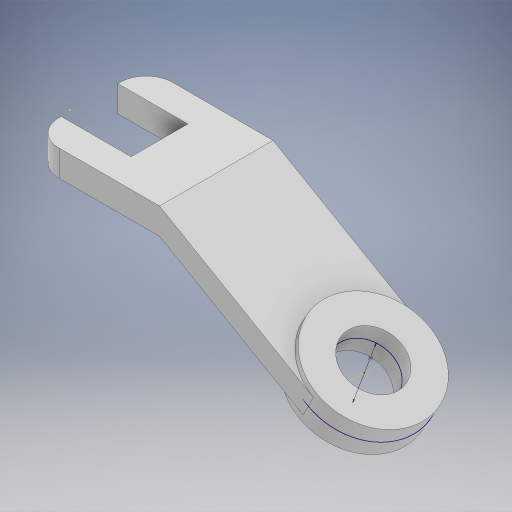
# Autodesk Inventor part: LE-1.4
Saved by Autodesk Inventor 2024 (Build 280153000, 153)
## iProperties
Created: 2024-01-25
Part Number: LE-1.4
Material: Generic
Document SubType Name: Modeling
Designer: Alex
Density: 1 g/cm^3
Appearance: Default
Author: Alex
Autodesk Inventor part; units mm, degrees
ref_plane "YZ Plane" through (0, 0, 0) normal (1, 0, 0) x (0, 1, 0)
ref_plane "XZ Plane" through (0, 0, 0) normal (0, 1, 0) x (-1, 0, 0)
sketch "Sketch1" plane through (0, 0, 0) normal (0, 0, 1) x (1, 0, 0)
  line L0 (0, 0) -> (58, 0)
  line L1 (58, 0) -> (58, 12)
  line L2 (58, 12) -> (0, 12)
  line L3 (0, 12) -> (0, 0)
  line L4 (58, 12) -> (36.0591, 24.6676) construction
  line L5 (58, 12) -> (129.0141, -29)
  line L6 (58, 12) -> (140, 12) construction
  line L7 (58, 0) -> (123.8179, -38)
  line L8 (58, 0) -> (134, 0) construction
  line L9 (123.8179, -38) -> (128.4714, -28.6867)
  dimension "d0" = 58
  dimension "d1" = 12
  dimension "d2" = 30
  dimension "d3" = 82
  dimension "d4" = 30
  dimension "d5" = 30
  dimension "d6" = 93.45
  dimension "d7" = 127.746
  dimension "d8" = 106.5151
  constraints: 20 end point, 3 horizontal, 2 equal length, 2 parallel, 1 perpendicular, 1 point on line
  measures "d0" distance of L2.end L1.end
  measures "d1" distance of L1.end L0.end
  measures "d2" angle of L2 L4
  measures "d3" distance of L1.end L5.end
  measures "d4" angle of L5 L6
  measures "d5" angle of L7 L8
  measures "d6" angle of L9 L5
  measures "d7" distance from line of L0.start L9
  measures "d8" distance from line of L4.end L9
extrude "Extrusion1" add sketch "Sketch1" against normal blind 52
ref_plane "Work Plane1" through (125.8734, -33.1867, 0) normal (0.5, 0.866, 0) x (0.866, -0.5, 0)
sketch "Sketch3" plane through (125.8734, -33.1867, 0) normal (0.5, 0.866, 0) x (0.866, -0.5, 0)
  line L0 (0, 0) -> (0, 52) construction
  circle A0 centre (0, 26) radius 26
  circle A1 centre (0, 26) radius 13
  point P0 (-125.6029, 0)
  dimension "d12" = 26
  constraints: 1 centre point, 1 coincident, 1 midpoint, 1 vertical alignment, 2 other
  measures "d12" diameter of A1
extrude "Extrusion2" add sketch "Sketch3" along normal mid plane 16
extrude "Extrusion3" cut sketch "Sketch3" along normal through all both and the other way through all contours A1
sketch "Sketch4" plane through (0, 12, 0) normal (0, 1, 0) x (1, 0, 0)
  line L0 (0, 0) -> (0, 52) projected
  line L1 (0, 26) -> (0, 39)
  line L2 (0, 39) -> (32, 39)
  line L3 (32, 39) -> (32, 13)
  line L4 (32, 13) -> (0, 13)
  line L5 (0, 13) -> (0, 39)
  dimension "d17" = 13
  dimension "d18" = 32
  dimension "d19" = 26
  constraints: 10 end point, 2 parallel, 1 horizontal, 1 midpoint, 1 perpendicular, 1 point on line
  measures "d17" distance of L1.start L1.end
  measures "d18" distance of L3.end L4.end
  measures "d19" distance of L2.end L3.end
extrude "Extrusion4" cut sketch "Sketch4" against normal through all
fillet "Fillet1" radius 12 2 edges at (0, 6, 0) (0, 6, -52)
body "Solid1"
